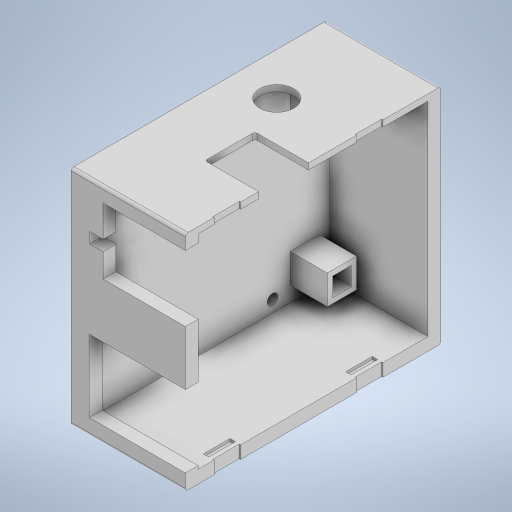
# Autodesk Inventor part: Enclosure_Top_v2
Saved by Autodesk Inventor 2023 (Build 270158030, 158C)
## iProperties
Created: 2023-12-07
Part Number: Enclosure_Top_v2
Material: Generic
Document SubType Name: Sheet Metal
Designer: Fabian
Density: 1 g/cm^3
Sheet Metal Rule: Default_mm
Appearance: Default
Author: Fabian
Autodesk Inventor part; units mm, degrees
ref_plane "YZ Plane" through (0, 0, 0) normal (1, 0, 0) x (0, 1, 0)
ref_plane "XZ Plane" through (0, 0, 0) normal (0, 1, 0) x (-1, 0, 0)
ref_plane "XY Plane" through (0, 0, 0) normal (0, 0, 1) x (1, 0, 0)
sketch "Sketch1" plane through (0, 0, 0) normal (1, 0, 0) x (0, 1, 0)
  line L0 (10.2141, 17.9541) -> (-31.7859, 17.9541)
  line L1 (-31.7859, 17.9541) -> (-31.7859, -30.1559)
  line L2 (-31.7859, -30.1559) -> (10.2141, -30.1559)
  line L3 (10.2141, -30.1559) -> (10.2141, 17.9541)
  point P0 (0, 0)
  dimension "d0" = 42
  dimension "d1" = 48.11
  constraints: 8 end point, 2 parallel, 1 horizontal, 1 perpendicular
  measures "d0" distance of L2.end L1.end
  measures "d1" distance of L1.end L0.end
extrude "BasePlate" add sketch "Sketch1" along normal blind 3
sketch "Sketch3" plane through (3, 0, 0) normal (1, 0, 0) x (0, 0, -1)
  line L0 (30.1559, 10.2141) -> (-17.9541, 10.2141) projected
  line L1 (-17.9541, -31.7859) -> (30.1559, -31.7859) projected
  line L2 (-17.9541, 10.2141) -> (30.1559, 10.2141)
  line L3 (30.1559, 10.2141) -> (30.1559, -31.7859)
  line L4 (30.1559, -31.7859) -> (-17.9541, -31.7859)
  line L5 (-17.9541, -31.7859) -> (-17.9541, 10.2141)
  line L6 (-15.5541, 9.0441) -> (27.7559, 9.0441)
  line L7 (27.7559, 9.0441) -> (27.7559, -29.3859)
  line L8 (27.7559, -29.3859) -> (-15.5541, -29.3859)
  line L9 (-15.5541, -29.3859) -> (-15.5541, 9.0441)
  point P0 (0, 0)
  point P1 (-17.9541, -10.7859)
  dimension "d4" = 1.17
  dimension "d5" = 2.4
  dimension "d6" = 2.4
  dimension "d7" = 2.4
  constraints: 16 end point, 4 parallel, 2 horizontal, 2 perpendicular, 1 midpoint
  measures "d4" distance between parallel lines of L0 L6
  measures "d5" distance between parallel lines of L1 L8
  measures "d6" distance from line of point (-17.954, -10.786) L9
  measures "d7" distance between parallel lines of L3 L7
extrude "Walls" add sketch "Sketch3" along normal blind 18.5
sketch "Sketch4" plane through (21.5, 0, 0) normal (1, 0, 0) x (0, 0, -1)
  line L0 (30.1559, 10.2141) -> (-17.9541, 10.2141) projected
  line L1 (-15.5541, 9.0441) -> (27.7559, 9.0441) projected
  line L2 (-4.1541, 10.2141) -> (5.2459, 10.2141)
  line L3 (5.2459, 10.2141) -> (5.2459, 9.0441)
  line L4 (5.2459, 9.0441) -> (-4.1541, 9.0441)
  line L5 (-4.1541, 9.0441) -> (-4.1541, 10.2141)
  line L6 (-17.9541, 10.2141) -> (-17.9541, -31.7859) projected
  point P0 (0, 0)
  point P1 (-4.1541, 9.6291)
  point P2 (5.2459, 10.2141)
  dimension "d10" = 9.4
  dimension "d11" = 13.8
  constraints: 8 end point, 2 parallel, 2 point on line, 1 horizontal, 1 midpoint, 1 perpendicular
  measures "d10" distance of L3.end L4.end
  measures "d11" distance from line of point (-4.154, 9.629) L6
extrude "USB-C" cut sketch "Sketch4" against normal blind 10.1
sketch "Sketch5" plane through (21.5, 0, 0) normal (1, 0, 0) x (0, 0, -1)
  line L0 (-17.9541, 10.2141) -> (-17.9541, -31.7859) projected
  line L1 (-15.5541, -29.3859) -> (-15.5541, 9.0441) projected
  line L2 (-17.9541, -4.8859) -> (-15.5541, -4.8859)
  line L3 (-15.5541, -4.8859) -> (-15.5541, 7.5141)
  line L4 (-15.5541, 7.5141) -> (-17.9541, 7.5141)
  line L5 (-17.9541, 7.5141) -> (-17.9541, -4.8859)
  line L6 (-4.1541, 10.2141) -> (-17.9541, 10.2141) projected
  point P0 (0, 0)
  point P1 (-16.7541, 7.5141)
  point P2 (-17.9541, 7.5141)
  point P3 (-15.5541, -4.8859)
  dimension "d14" = 12.4
  dimension "d15" = 2.7
  constraints: 8 end point, 2 parallel, 2 point on line, 1 horizontal, 1 midpoint, 1 perpendicular
  measures "d14" distance of L3.end L2.end
  measures "d15" distance from line of L6 point (-16.754, 7.514)
extrude "PowerConnector1" cut sketch "Sketch5" against normal blind 15.5
sketch "Sketch6" plane through (6, 0, 0) normal (1, 0, 0) x (0, 0, -1)
  line L0 (-17.9541, 10.2141) -> (-17.9541, -31.7859) projected
  line L1 (-17.9541, -0.3859) -> (-15.5541, -0.3859)
  line L2 (-15.5541, -0.3859) -> (-15.5541, 1.6141)
  line L3 (-15.5541, 1.6141) -> (-17.9541, 1.6141)
  line L4 (-17.9541, 1.6141) -> (-17.9541, -0.3859)
  line L5 (-17.9541, 7.5141) -> (-15.5541, 7.5141) projected
  point P0 (0, 0)
  dimension "d18" = 2.4
  dimension "d19" = 2
  dimension "d20" = 5.9
  constraints: 8 end point, 2 parallel, 1 horizontal, 1 perpendicular, 1 point on line
  measures "d18" distance of L3.end L2.end
  measures "d19" distance of L1.end L2.end
  measures "d20" distance between parallel lines of L5 L3
extrude "PowerConnector2" cut sketch "Sketch6" against normal blind 2.5
sketch "Sketch8" plane through (21.5, 0, 0) normal (1, 0, 0) x (0, 0, -1)
  line L0 (-17.9541, 10.2141) -> (-17.9541, -31.7859) projected
  line L1 (-15.5541, 9.0441) -> (-15.5541, -29.3859) projected
  line L2 (-17.9541, -28.7859) -> (-15.5541, -28.7859)
  line L3 (-15.5541, -28.7859) -> (-15.5541, -15.1859)
  line L4 (-15.5541, -15.1859) -> (-17.9541, -15.1859)
  line L5 (-17.9541, -15.1859) -> (-17.9541, -28.7859)
  line L6 (-17.9541, -31.7859) -> (30.1559, -31.7859) projected
  point P0 (0, 0)
  dimension "d23" = 13.6
  dimension "d24" = 3
  constraints: 8 end point, 2 parallel, 2 point on line, 1 horizontal, 1 perpendicular
  measures "d23" distance of L3.end L2.end
  measures "d24" distance between parallel lines of L6 L2
extrude "RJ-12" cut sketch "Sketch8" against normal blind 18.1
fillet "Fillet1" radius 0.5 4 edges at (10.75, 10.2141, 17.9541) (10.75, -31.7859, 17.9541) (10.75, 10.2141, -30.1559) (10.75, -31.7859, -30.1559)
sketch "Sketch9" plane through (0, 0, 0) normal (-1, 0, 0) x (0, 0, 1)
  line L0 (-24.8059, -25.5359) -> (-21.3059, -25.5359)
  line L1 (-21.3059, -25.5359) -> (-21.3059, -22.0359)
  line L2 (-21.3059, -22.0359) -> (-24.8059, -22.0359)
  line L3 (-24.8059, -22.0359) -> (-24.8059, -25.5359)
  line L4 (-30.1559, -31.2859) -> (-30.1559, 9.7141) projected
  line L5 (17.4541, -31.7859) -> (-29.6559, -31.7859) projected
  point P0 (0, 0)
  point P1 (-24.8059, -23.7859)
  dimension "d28" = 3.5
  dimension "d29" = 3.5
  dimension "d30" = 5.35
  dimension "d31" = 6.25
  constraints: 8 end point, 2 parallel, 1 horizontal, 1 midpoint, 1 perpendicular
  measures "d28" distance of L2.end L1.end
  measures "d29" distance of L1.end L0.end
  measures "d30" distance from line of L4 point (-24.806, -23.786)
  measures "d31" distance between parallel lines of L5 L0
extrude "ZBButton" cut sketch "Sketch9" against normal blind 3
sketch "Sketch10" plane through (0, 0, 0) normal (-1, 0, 0) x (0, 0, 1)
  line L0 (-24.8059, 0.6641) -> (-21.3059, 0.6641)
  line L1 (-21.3059, 0.6641) -> (-21.3059, 4.1641)
  line L2 (-21.3059, 4.1641) -> (-24.8059, 4.1641)
  line L3 (-24.8059, 4.1641) -> (-24.8059, 0.6641)
  line L4 (-30.1559, -31.2859) -> (-30.1559, 9.7141) projected
  line L5 (-29.6559, 10.2141) -> (17.4541, 10.2141) projected
  point P0 (0, 0)
  point P1 (-24.8059, 2.4141)
  dimension "d34" = 3.5
  dimension "d35" = 3.5
  dimension "d36" = 5.35
  dimension "d37" = 6.05
  constraints: 8 end point, 2 parallel, 1 horizontal, 1 midpoint, 1 perpendicular
  measures "d34" distance of L2.end L1.end
  measures "d35" distance of L1.end L0.end
  measures "d36" distance from line of L4 point (-24.806, 2.414)
  measures "d37" distance between parallel lines of L5 L2
extrude "ResetButton" cut sketch "Sketch10" against normal blind 3
sketch "Sketch11" plane through (3, 0, 0) normal (1, 0, 0) x (0, 0, -1)
  line L0 (25.8059, 5.1641) -> (20.3059, 5.1641)
  line L1 (20.3059, 5.1641) -> (20.3059, -0.3359)
  line L2 (20.3059, -0.3359) -> (25.8059, -0.3359)
  line L3 (25.8059, -0.3359) -> (25.8059, 5.1641)
  line L4 (21.3059, 4.1641) -> (24.8059, 4.1641) projected
  line L5 (24.8059, 4.1641) -> (24.8059, 0.6641) projected
  line L6 (25.8059, -21.0359) -> (20.3059, -21.0359)
  line L7 (20.3059, -21.0359) -> (20.3059, -26.5359)
  line L8 (20.3059, -26.5359) -> (25.8059, -26.5359)
  line L9 (25.8059, -26.5359) -> (25.8059, -21.0359)
  line L10 (24.8059, -22.0359) -> (24.8059, -25.5359) projected
  line L11 (21.3059, -22.0359) -> (24.8059, -22.0359) projected
  line L12 (24.8059, 0.6641) -> (21.3059, 0.6641) projected
  line L13 (24.8059, 4.1641) -> (21.3059, 4.1641)
  line L14 (21.3059, 4.1641) -> (21.3059, 0.6641)
  line L15 (21.3059, 0.6641) -> (24.8059, 0.6641)
  line L16 (24.8059, 0.6641) -> (24.8059, 4.1641)
  line L17 (21.3059, -25.5359) -> (21.3059, -22.0359) projected
  line L18 (24.8059, -22.0359) -> (21.3059, -22.0359)
  line L19 (21.3059, -22.0359) -> (21.3059, -25.5359)
  line L20 (21.3059, -25.5359) -> (24.8059, -25.5359)
  line L21 (24.8059, -25.5359) -> (24.8059, -22.0359)
  point P0 (0, 0)
  point P1 (23.0559, -22.0359)
  dimension "d40" = 5.5
  dimension "d41" = 5.5
  dimension "d42" = 1
  dimension "d43" = 1
  dimension "d44" = 5.5
  dimension "d45" = 5.5
  dimension "d46" = 1
  dimension "d47" = 1
  constraints: 32 end point, 8 parallel, 4 horizontal, 4 perpendicular, 1 midpoint
  measures "d40" distance of L2.end L1.end
  measures "d41" distance of L1.end L0.end
  measures "d42" distance between parallel lines of L4 L0
  measures "d43" distance between parallel lines of L3 L5
  measures "d44" distance of L8.end L7.end
  measures "d45" distance of L7.end L6.end
  measures "d46" distance between parallel lines of L9 L10
  measures "d47" distance from line of point (23.056, -22.036) L6
extrude "ButtonFuehrung" add sketch "Sketch11" along normal blind 7
sketch "Sketch12" plane through (0, 0, 0) normal (-1, 0, 0) x (0, 0, 1)
  circle A0 centre (-16.9559, -27.1859) radius 1
  line L0 (17.4541, -31.7859) -> (-29.6559, -31.7859) projected
  line L1 (-30.1559, -31.2859) -> (-30.1559, 9.7141) projected
  point P0 (0, 0)
  dimension "d50" = 2
  dimension "d51" = 4.6
  dimension "d52" = 13.2
  constraints: 1 centre point
  measures "d50" diameter of A0
  measures "d51" distance from line of L0 A0.centre
  measures "d52" distance from line of L1 A0.centre
extrude "LED" cut sketch "Sketch12" against normal blind 3
sketch "Sketch13" plane through (11.4, 10.2141, 4.1541) normal (0, 1, 0) x (1, 0, 0)
  circle A0 centre (-3.4, 16.91) radius 3.2
  line L0 (-11.4, 33.81) -> (-11.4, -13.3) projected
  line L1 (10.1, 34.31) -> (-11.4, 34.31) projected
  point P0 (-11.4, 4.1541)
  dimension "d55" = 6.4
  dimension "d56" = 8
  dimension "d57" = 17.4
  constraints: 1 centre point
  measures "d55" diameter of A0
  measures "d56" distance from line of L0 A0.centre
  measures "d57" distance from line of L1 A0.centre
extrude "Antenna" cut sketch "Sketch13" against normal blind 2
sketch "Sketch14" plane through (3, 9.0441, -27.7559) normal (0, -1, 0) x (1, 0, 0)
  line L0 (17.5, 40.31) -> (16.5, 40.31)
  line L1 (16.5, 40.31) -> (16.5, 35.31)
  line L2 (16.5, 35.31) -> (17.5, 35.31)
  line L3 (17.5, 35.31) -> (17.5, 40.31)
  line L4 (18.5, 43.31) -> (18.5, 31.91) projected
  point P0 (-3, 27.7559)
  point P1 (17.5, 37.81)
  dimension "d60" = 1
  dimension "d61" = 5
  dimension "d62" = 1
  dimension "d63" = 5.5
  constraints: 8 end point, 2 parallel, 1 horizontal, 1 midpoint, 1 perpendicular
  measures "d60" distance of L2.end L1.end
  measures "d61" distance of L1.end L0.end
  measures "d62" distance between parallel lines of L4 L3
  measures "d63" vertical distance of L4.start point (17.5, 37.81)
extrude "Extrusion12" cut sketch "Sketch14" against normal blind 0.5
sketch "Sketch15" plane through (3, 9.0441, -27.7559) normal (0, -1, 0) x (1, 0, 0)
  line L0 (17.5, 13.5) -> (16.5, 13.5)
  line L1 (16.5, 13.5) -> (16.5, 8.5)
  line L2 (16.5, 8.5) -> (17.5, 8.5)
  line L3 (17.5, 8.5) -> (17.5, 13.5)
  line L4 (18.5, 22.51) -> (18.5, 0) projected
  line L5 (0, 0) -> (18.5, 0) projected
  point P0 (-3, 27.7559)
  point P1 (17.5, 11)
  dimension "d66" = 1
  dimension "d67" = 5
  dimension "d68" = 1
  dimension "d69" = 11
  constraints: 8 end point, 2 parallel, 1 horizontal, 1 midpoint, 1 perpendicular
  measures "d66" distance of L2.end L1.end
  measures "d67" distance of L1.end L0.end
  measures "d68" distance from line of L4 point (17.5, 11)
  measures "d69" distance from line of L5 point (17.5, 11)
extrude "Extrusion13" cut sketch "Sketch15" against normal blind 0.5
sketch "Sketch16" plane through (3, -29.3859, 15.5541) normal (0, 1, 0) x (1, 0, 0)
  line L0 (17.5, 8) -> (16.5, 8)
  line L1 (16.5, 8) -> (16.5, 3)
  line L2 (16.5, 3) -> (17.5, 3)
  line L3 (17.5, 3) -> (17.5, 8)
  line L4 (18.5, 43.31) -> (18.5, 0) projected
  line L5 (0, 0) -> (18.5, 0) projected
  point P0 (-3, 15.5541)
  point P1 (17.5, 5.5)
  dimension "d72" = 1
  dimension "d73" = 5
  dimension "d74" = 1
  dimension "d75" = 5.5
  constraints: 8 end point, 2 parallel, 1 horizontal, 1 midpoint, 1 perpendicular
  measures "d72" distance of L2.end L1.end
  measures "d73" distance of L1.end L0.end
  measures "d74" distance between parallel lines of L4 L3
  measures "d75" distance from line of L5 point (17.5, 5.5)
extrude "Extrusion14" cut sketch "Sketch16" against normal blind 0.5
sketch "Sketch17" plane through (3, -29.3859, 15.5541) normal (0, 1, 0) x (1, 0, 0)
  line L0 (17.5, 34.81) -> (16.5, 34.81)
  line L1 (16.5, 34.81) -> (16.5, 29.81)
  line L2 (16.5, 29.81) -> (17.5, 29.81)
  line L3 (17.5, 29.81) -> (17.5, 34.81)
  line L4 (18.5, 43.31) -> (18.5, 0) projected
  line L5 (0, 43.31) -> (18.5, 43.31) projected
  point P0 (-3, 15.5541)
  point P1 (17.5, 32.31)
  dimension "d78" = 1
  dimension "d79" = 5
  dimension "d80" = 1
  dimension "d81" = 11
  constraints: 8 end point, 2 parallel, 1 horizontal, 1 midpoint, 1 perpendicular
  measures "d78" distance of L2.end L1.end
  measures "d79" distance of L1.end L0.end
  measures "d80" distance between parallel lines of L4 L3
  measures "d81" distance from line of L5 point (17.5, 32.31)
extrude "Extrusion15" cut sketch "Sketch17" against normal blind 0.5
fillet "Fillet2" radius 0.5 2 edges at (11.4, 9.6291, -5.2459) (11.4, 9.6291, 4.1541)
sketch "Sketch18" plane through (0, 0, 0) normal (-1, 0, 0) x (0, 0, 1)
  line L0 (-25.0559, 8.7746) -> (-25.0559, -4.7256) construction
  line L1 (-25.0559, -4.7256) -> (-29.2477, -4.7256) construction
  line L2 (-29.2477, -4.7256) -> (-29.2477, 8.7746) construction
  line L3 (-29.2477, 8.7746) -> (-25.0559, 8.7746) construction
  line L4 (-25.0559, -16.0398) -> (-25.0559, -32.4133) construction
  line L5 (-25.0559, -32.4133) -> (-30.1806, -32.4133) construction
  line L6 (-30.1806, -32.4133) -> (-30.1806, -16.0398) construction
  line L7 (-30.1806, -16.0398) -> (-25.0559, -16.0398) construction
  line L8 (-24.8059, -25.5359) -> (-24.8059, -22.0359) projected
  line L9 (-24.8059, 0.6641) -> (-24.8059, 4.1641) projected
  line L10 (-28.5559, 5.7114) -> (-28.5559, 6.3155)
  line L11 (-28.5559, 6.3155) -> (-27.1633, 7.4217)
  line L12 (-27.1633, 7.4217) -> (-27.1633, 7.9549)
  line L13 (-27.1633, 7.9549) -> (-28.5559, 7.9549)
  line L14 (-28.5559, 7.9549) -> (-28.5559, 8.42)
  line L15 (-28.5559, 8.42) -> (-25.0559, 8.42)
  line L16 (-25.0559, 8.42) -> (-25.0559, 7.5181)
  spline S0 degree 2 poles (-25.0559, 7.5181) (-25.0559, 7.2174) (-25.1212, 6.8119) (-25.2403, 6.6275) knots 0 0 0 1 2 2 2
  spline S1 degree 2 poles (-25.2403, 6.6275) (-25.3594, 6.4431) (-25.731, 6.2304) (-26.0061, 6.2304) knots 0 0 0 1 2 2 2
  spline S2 degree 2 poles (-26.0061, 6.2304) (-26.389, 6.2304) (-26.908, 6.6218) (-27.0328, 6.9565) knots 0 0 0 1 2 2 2
  line L17 (-27.0328, 6.9565) -> (-28.5559, 5.7114)
  spline S3 degree 2 poles (-26.043, 6.7154) (-25.8898, 6.7154) (-25.6544, 6.8232) (-25.5778, 6.9367) knots 0 0 0 1 2 2 2
  spline S4 degree 2 poles (-25.5778, 6.9367) (-25.5126, 7.0359) (-25.4587, 7.2997) (-25.4587, 7.4926) knots 0 0 0 1 2 2 2
  line L18 (-25.4587, 7.4926) -> (-25.4587, 7.9549)
  line L19 (-25.4587, 7.9549) -> (-26.7747, 7.9549)
  line L20 (-26.7747, 7.9549) -> (-26.7747, 7.5465)
  spline S5 degree 2 poles (-26.7747, 7.5465) (-26.7747, 7.3451) (-26.7038, 7.0246) (-26.5932, 6.914) knots 0 0 0 1 2 2 2
  spline S6 degree 2 poles (-26.5932, 6.914) (-26.4968, 6.8119) (-26.2245, 6.7154) (-26.043, 6.7154) knots 0 0 0 1 2 2 2
  spline S7 degree 2 poles (-28.6155, 4.3272) (-28.6155, 4.9569) (-27.9093, 5.649) (-27.2569, 5.649) knots 0 0 0 1 2 2 2
  spline S8 degree 2 poles (-27.2569, 5.649) (-26.6159, 5.649) (-25.8558, 4.9768) (-25.8558, 4.435) knots 0 0 0 1 2 2 2
  spline S9 degree 2 poles (-25.8558, 4.435) (-25.8558, 4.1911) (-25.9976, 3.8139) (-26.1479, 3.6749) knots 0 0 0 1 2 2 2
  spline S10 degree 2 poles (-26.1479, 3.6749) (-26.2982, 3.5331) (-26.7322, 3.3828) (-27.047, 3.3828) knots 0 0 0 1 2 2 2
  line L21 (-27.047, 3.3828) -> (-27.2881, 3.3828)
  line L22 (-27.2881, 3.3828) -> (-27.2881, 5.2008)
  spline S11 degree 2 poles (-27.2881, 5.2008) (-27.7448, 5.2008) (-28.2298, 4.7414) (-28.2298, 4.3329) knots 0 0 0 1 2 2 2
  spline S12 degree 2 poles (-28.2298, 4.3329) (-28.2298, 4.1883) (-28.1645, 3.9075) (-28.1135, 3.794) knots 0 0 0 1 2 2 2
  spline S13 degree 2 poles (-28.1135, 3.794) (-28.0568, 3.6749) (-27.9575, 3.5104) (-27.9121, 3.4565) knots 0 0 0 1 2 2 2
  line L23 (-27.9121, 3.4565) -> (-27.9121, 3.431)
  line L24 (-27.9121, 3.431) -> (-28.3943, 3.431)
  spline S14 degree 2 poles (-28.3943, 3.431) (-28.4255, 3.5076) (-28.5162, 3.7401) (-28.5418, 3.8309) knots 0 0 0 1 2 2 2
  spline S15 degree 2 poles (-28.5418, 3.8309) (-28.5786, 3.9585) (-28.6155, 4.1684) (-28.6155, 4.3272) knots 0 0 0 1 2 2 2
  spline S16 degree 2 poles (-26.9506, 3.8139) (-26.7719, 3.8196) (-26.511, 3.8933) (-26.423, 3.9642) knots 0 0 0 1 2 2 2
  spline S17 degree 2 poles (-26.423, 3.9642) (-26.3238, 4.0408) (-26.2188, 4.2819) (-26.2188, 4.4606) knots 0 0 0 1 2 2 2
  spline S18 degree 2 poles (-26.2188, 4.4606) (-26.2188, 4.6364) (-26.3238, 4.8832) (-26.4259, 4.9853) knots 0 0 0 1 2 2 2
  spline S19 degree 2 poles (-26.4259, 4.9853) (-26.5308, 5.0845) (-26.7833, 5.1867) (-26.9506, 5.2008) knots 0 0 0 1 2 2 2
  line L25 (-26.9506, 5.2008) -> (-26.9506, 3.8139)
  spline S20 degree 2 poles (-28.6183, 2.2255) (-28.6183, 2.4893) (-28.4765, 2.946) (-28.3971, 3.0963) knots 0 0 0 1 2 2 2
  line L26 (-28.3971, 3.0963) -> (-27.9008, 3.0963)
  line L27 (-27.9008, 3.0963) -> (-27.9008, 3.0736)
  spline S21 degree 2 poles (-27.9008, 3.0736) (-27.9461, 3.0169) (-28.0539, 2.8637) (-28.1135, 2.7361) knots 0 0 0 1 2 2 2
  spline S22 degree 2 poles (-28.1135, 2.7361) (-28.1674, 2.6255) (-28.2468, 2.3532) (-28.2468, 2.2085) knots 0 0 0 1 2 2 2
  spline S23 degree 2 poles (-28.2468, 2.2085) (-28.2468, 2.1036) (-28.1986, 1.8625) (-28.1589, 1.8058) knots 0 0 0 1 2 2 2
  spline S24 degree 2 poles (-28.1589, 1.8058) (-28.105, 1.7235) (-27.983, 1.6498) (-27.8582, 1.6498) knots 0 0 0 1 2 2 2
  spline S25 degree 2 poles (-27.8582, 1.6498) (-27.7022, 1.6498) (-27.5405, 1.82) (-27.4867, 2.0384) knots 0 0 0 1 2 2 2
  spline S26 degree 2 poles (-27.4867, 2.0384) (-27.4668, 2.1234) (-27.4101, 2.3957) (-27.3789, 2.512) knots 0 0 0 1 2 2 2
  spline S27 degree 2 poles (-27.3789, 2.512) (-27.2909, 2.8127) (-26.9279, 3.0849) (-26.6698, 3.0849) knots 0 0 0 1 2 2 2
  spline S28 degree 2 poles (-26.6698, 3.0849) (-26.3124, 3.0849) (-25.8671, 2.5489) (-25.8671, 2.1064) knots 0 0 0 1 2 2 2
  spline S29 degree 2 poles (-25.8671, 2.1064) (-25.8671, 1.888) (-25.9749, 1.4456) (-26.0572, 1.2952) knots 0 0 0 1 2 2 2
  line L28 (-26.0572, 1.2952) -> (-26.5308, 1.2952)
  line L29 (-26.5308, 1.2952) -> (-26.5308, 1.3179)
  spline S30 degree 2 poles (-26.5308, 1.3179) (-26.3947, 1.4881) (-26.2387, 1.9022) (-26.2387, 2.1149) knots 0 0 0 1 2 2 2
  spline S31 degree 2 poles (-26.2387, 2.1149) (-26.2387, 2.3333) (-26.423, 2.634) (-26.6074, 2.634) knots 0 0 0 1 2 2 2
  spline S32 degree 2 poles (-26.6074, 2.634) (-26.7747, 2.634) (-26.9364, 2.4553) (-26.9875, 2.2567) knots 0 0 0 1 2 2 2
  spline S33 degree 2 poles (-26.9875, 2.2567) (-27.013, 2.1603) (-27.064, 1.9164) (-27.0952, 1.7831) knots 0 0 0 1 2 2 2
  spline S34 degree 2 poles (-27.0952, 1.7831) (-27.169, 1.4938) (-27.5065, 1.1988) (-27.7986, 1.1988) knots 0 0 0 1 2 2 2
  spline S35 degree 2 poles (-27.7986, 1.1988) (-27.9688, 1.1988) (-28.2695, 1.3321) (-28.3801, 1.4626) knots 0 0 0 1 2 2 2
  spline S36 degree 2 poles (-28.3801, 1.4626) (-28.4964, 1.6016) (-28.6183, 1.9561) (-28.6183, 2.2255) knots 0 0 0 1 2 2 2
  spline S37 degree 2 poles (-28.6155, -0.3527) (-28.6155, 0.277) (-27.9093, 0.9691) (-27.2569, 0.9691) knots 0 0 0 1 2 2 2
  spline S38 degree 2 poles (-27.2569, 0.9691) (-26.6159, 0.9691) (-25.8558, 0.2969) (-25.8558, -0.2449) knots 0 0 0 1 2 2 2
  spline S39 degree 2 poles (-25.8558, -0.2449) (-25.8558, -0.4888) (-25.9976, -0.866) (-26.1479, -1.005) knots 0 0 0 1 2 2 2
  spline S40 degree 2 poles (-26.1479, -1.005) (-26.2982, -1.1468) (-26.7322, -1.2971) (-27.047, -1.2971) knots 0 0 0 1 2 2 2
  line L30 (-27.047, -1.2971) -> (-27.2881, -1.2971)
  line L31 (-27.2881, -1.2971) -> (-27.2881, 0.5209)
  spline S41 degree 2 poles (-27.2881, 0.5209) (-27.7448, 0.5209) (-28.2298, 0.0614) (-28.2298, -0.347) knots 0 0 0 1 2 2 2
  spline S42 degree 2 poles (-28.2298, -0.347) (-28.2298, -0.4916) (-28.1645, -0.7724) (-28.1135, -0.8859) knots 0 0 0 1 2 2 2
  spline S43 degree 2 poles (-28.1135, -0.8859) (-28.0568, -1.005) (-27.9575, -1.1695) (-27.9121, -1.2234) knots 0 0 0 1 2 2 2
  line L32 (-27.9121, -1.2234) -> (-27.9121, -1.2489)
  line L33 (-27.9121, -1.2489) -> (-28.3943, -1.2489)
  spline S44 degree 2 poles (-28.3943, -1.2489) (-28.4255, -1.1723) (-28.5162, -0.9398) (-28.5418, -0.849) knots 0 0 0 1 2 2 2
  spline S45 degree 2 poles (-28.5418, -0.849) (-28.5786, -0.7214) (-28.6155, -0.5115) (-28.6155, -0.3527) knots 0 0 0 1 2 2 2
  spline S46 degree 2 poles (-26.9506, -0.866) (-26.7719, -0.8604) (-26.511, -0.7866) (-26.423, -0.7157) knots 0 0 0 1 2 2 2
  spline S47 degree 2 poles (-26.423, -0.7157) (-26.3238, -0.6391) (-26.2188, -0.398) (-26.2188, -0.2193) knots 0 0 0 1 2 2 2
  spline S48 degree 2 poles (-26.2188, -0.2193) (-26.2188, -0.0435) (-26.3238, 0.2033) (-26.4259, 0.3054) knots 0 0 0 1 2 2 2
  spline S49 degree 2 poles (-26.4259, 0.3054) (-26.5308, 0.4046) (-26.7833, 0.5067) (-26.9506, 0.5209) knots 0 0 0 1 2 2 2
  line L34 (-26.9506, 0.5209) -> (-26.9506, -0.866)
  spline S50 degree 2 poles (-28.607, -2.5394) (-28.607, -2.1792) (-28.1957, -1.7736) (-27.7504, -1.7736) knots 0 0 0 1 2 2 2
  line L35 (-27.7504, -1.7736) -> (-26.2954, -1.7736)
  line L36 (-26.2954, -1.7736) -> (-26.2954, -1.4758)
  line L37 (-26.2954, -1.4758) -> (-25.9295, -1.4758)
  line L38 (-25.9295, -1.4758) -> (-25.9295, -1.7736)
  line L39 (-25.9295, -1.7736) -> (-25.1751, -1.7736)
  line L40 (-25.1751, -1.7736) -> (-25.1751, -2.2161)
  line L41 (-25.1751, -2.2161) -> (-25.9295, -2.2161)
  line L42 (-25.9295, -2.2161) -> (-25.9295, -3.0301)
  line L43 (-25.9295, -3.0301) -> (-26.2954, -3.0301)
  line L44 (-26.2954, -3.0301) -> (-26.2954, -2.2161)
  line L45 (-26.2954, -2.2161) -> (-27.5462, -2.2161)
  spline S51 degree 2 poles (-27.5462, -2.2161) (-27.7448, -2.2161) (-27.9632, -2.2303) (-28.0568, -2.2785) knots 0 0 0 1 2 2 2
  spline S52 degree 2 poles (-28.0568, -2.2785) (-28.139, -2.3182) (-28.2213, -2.4969) (-28.2213, -2.6501) knots 0 0 0 1 2 2 2
  spline S53 degree 2 poles (-28.2213, -2.6501) (-28.2213, -2.7578) (-28.156, -2.9592) (-28.1362, -3.0046) knots 0 0 0 1 2 2 2
  line L46 (-28.1362, -3.0046) -> (-28.1362, -3.0301)
  line L47 (-28.1362, -3.0301) -> (-28.5333, -3.0301)
  spline S54 degree 2 poles (-28.5333, -3.0301) (-28.5673, -2.9053) (-28.607, -2.6501) (-28.607, -2.5394) knots 0 0 0 1 2 2 2
  line L48 (-28.5786, -18.6265) -> (-28.5786, -16.1816)
  line L49 (-28.5786, -16.1816) -> (-28.1447, -16.1816)
  line L50 (-28.1447, -16.1816) -> (-25.4927, -18.0535)
  line L51 (-25.4927, -18.0535) -> (-25.4927, -16.2667)
  line L52 (-25.4927, -16.2667) -> (-25.0786, -16.2667)
  line L53 (-25.0786, -16.2667) -> (-25.0786, -18.5783)
  line L54 (-25.0786, -18.5783) -> (-25.4984, -18.5783)
  line L55 (-25.4984, -18.5783) -> (-28.1645, -16.6864)
  line L56 (-28.1645, -16.6864) -> (-28.1645, -18.6265)
  line L57 (-28.1645, -18.6265) -> (-28.5786, -18.6265)
  line L58 (-28.5786, -19.5029) -> (-28.5786, -19.0604)
  line L59 (-28.5786, -19.0604) -> (-25.9522, -19.0604)
  line L60 (-25.9522, -19.0604) -> (-25.9522, -19.5029)
  line L61 (-25.9522, -19.5029) -> (-28.5786, -19.5029)
  line L62 (-25.5154, -19.5341) -> (-25.5154, -19.0321)
  line L63 (-25.5154, -19.0321) -> (-25.0559, -19.0321)
  line L64 (-25.0559, -19.0321) -> (-25.0559, -19.5341)
  line L65 (-25.0559, -19.5341) -> (-25.5154, -19.5341)
  spline S55 degree 2 poles (-28.9984, -20.246) (-29.0183, -20.2914) (-29.0807, -20.4644) (-29.1062, -20.575) knots 0 0 0 1 2 2 2
  spline S56 degree 2 poles (-29.1062, -20.575) (-29.1374, -20.697) (-29.1743, -20.904) (-29.1743, -21.026) knots 0 0 0 1 2 2 2
  spline S57 degree 2 poles (-29.1743, -21.026) (-29.1743, -21.2302) (-29.0665, -21.5138) (-28.97, -21.5933) knots 0 0 0 1 2 2 2
  spline S58 degree 2 poles (-28.97, -21.5933) (-28.8736, -21.6698) (-28.6212, -21.7294) (-28.4595, -21.7294) knots 0 0 0 1 2 2 2
  line L66 (-28.4595, -21.7294) -> (-28.2298, -21.7294)
  spline S59 degree 2 poles (-28.2298, -21.7294) (-28.3858, -21.5507) (-28.5333, -21.2075) (-28.5333, -20.9494) knots 0 0 0 1 2 2 2
  spline S60 degree 2 poles (-28.5333, -20.9494) (-28.5333, -20.5013) (-27.8667, -19.9709) (-27.2399, -19.9709) knots 0 0 0 1 2 2 2
  spline S61 degree 2 poles (-27.2399, -19.9709) (-26.9137, -19.9709) (-26.4089, -20.1552) (-26.2302, -20.3084) knots 0 0 0 1 2 2 2
  spline S62 degree 2 poles (-26.2302, -20.3084) (-26.0628, -20.4559) (-25.8785, -20.8615) (-25.8785, -21.077) knots 0 0 0 1 2 2 2
  spline S63 degree 2 poles (-25.8785, -21.077) (-25.8785, -21.2813) (-25.9749, -21.5791) (-26.0628, -21.7294) knots 0 0 0 1 2 2 2
  line L67 (-26.0628, -21.7294) -> (-25.9522, -21.7549)
  line L68 (-25.9522, -21.7549) -> (-25.9522, -22.1719)
  line L69 (-25.9522, -22.1719) -> (-28.278, -22.1719)
  spline S64 degree 2 poles (-28.278, -22.1719) (-28.9474, -22.1719) (-29.5713, -21.5904) (-29.5713, -20.992) knots 0 0 0 1 2 2 2
  spline S65 degree 2 poles (-29.5713, -20.992) (-29.5713, -20.7991) (-29.5089, -20.3963) (-29.4579, -20.2233) knots 0 0 0 1 2 2 2
  line L70 (-29.4579, -20.2233) -> (-28.9984, -20.2233)
  line L71 (-28.9984, -20.2233) -> (-28.9984, -20.246)
  line L72 (-27.8667, -21.7294) -> (-26.423, -21.7294)
  spline S66 degree 2 poles (-26.423, -21.7294) (-26.3436, -21.5649) (-26.2756, -21.2869) (-26.2756, -21.148) knots 0 0 0 1 2 2 2
  spline S67 degree 2 poles (-26.2756, -21.148) (-26.2756, -20.8133) (-26.7691, -20.4275) (-27.2314, -20.4275) knots 0 0 0 1 2 2 2
  spline S68 degree 2 poles (-27.2314, -20.4275) (-27.6682, -20.4275) (-28.1248, -20.7197) (-28.1248, -21.0487) knots 0 0 0 1 2 2 2
  spline S69 degree 2 poles (-28.1248, -21.0487) (-28.1248, -21.2217) (-27.9887, -21.5847) (-27.8667, -21.7294) knots 0 0 0 1 2 2 2
  spline S70 degree 2 poles (-27.5037, -25.2209) (-27.7646, -25.2209) (-28.1645, -25.0223) (-28.295, -24.8578) knots 0 0 0 1 2 2 2
  spline S71 degree 2 poles (-28.295, -24.8578) (-28.4482, -24.6593) (-28.5786, -24.2083) (-28.5786, -23.851) knots 0 0 0 1 2 2 2
  line L73 (-28.5786, -23.851) -> (-28.5786, -22.8469)
  line L74 (-28.5786, -22.8469) -> (-25.0786, -22.8469)
  line L75 (-25.0786, -22.8469) -> (-25.0786, -23.7744)
  spline S72 degree 2 poles (-25.0786, -23.7744) (-25.0786, -24.1488) (-25.1268, -24.5232) (-25.2204, -24.6933) knots 0 0 0 1 2 2 2
  spline S73 degree 2 poles (-25.2204, -24.6933) (-25.3197, -24.8834) (-25.6459, -25.0564) (-25.8671, -25.0564) knots 0 0 0 1 2 2 2
  spline S74 degree 2 poles (-25.8671, -25.0564) (-26.1139, -25.0564) (-26.5053, -24.7954) (-26.6159, -24.5657) knots 0 0 0 1 2 2 2
  line L76 (-26.6159, -24.5657) -> (-26.6329, -24.5657)
  spline S75 degree 2 poles (-26.6329, -24.5657) (-26.718, -24.8777) (-27.169, -25.2209) (-27.5037, -25.2209) knots 0 0 0 1 2 2 2
  spline S76 degree 2 poles (-27.5235, -24.7359) (-27.325, -24.7359) (-27.0697, -24.6224) (-26.979, -24.4523) knots 0 0 0 1 2 2 2
  spline S77 degree 2 poles (-26.979, -24.4523) (-26.9222, -24.3416) (-26.8882, -24.0807) (-26.8882, -23.8396) knots 0 0 0 1 2 2 2
  line L77 (-26.8882, -23.8396) -> (-26.8882, -23.3121)
  line L78 (-26.8882, -23.3121) -> (-28.1815, -23.3121)
  line L79 (-28.1815, -23.3121) -> (-28.1815, -23.6893)
  spline S78 degree 2 poles (-28.1815, -23.6893) (-28.1815, -23.9956) (-28.1248, -24.3473) (-28.0341, -24.4835) knots 0 0 0 1 2 2 2
  spline S79 degree 2 poles (-28.0341, -24.4835) (-27.9405, -24.6139) (-27.7079, -24.7359) (-27.5235, -24.7359) knots 0 0 0 1 2 2 2
  spline S80 degree 2 poles (-25.9324, -24.5714) (-25.8076, -24.5714) (-25.6204, -24.4863) (-25.5665, -24.3927) knots 0 0 0 1 2 2 2
  spline S81 degree 2 poles (-25.5665, -24.3927) (-25.5041, -24.2792) (-25.4757, -24.0041) (-25.4757, -23.7574) knots 0 0 0 1 2 2 2
  line L80 (-25.4757, -23.7574) -> (-25.4757, -23.3121)
  line L81 (-25.4757, -23.3121) -> (-26.4996, -23.3121)
  line L82 (-26.4996, -23.3121) -> (-26.4996, -23.8396)
  spline S82 degree 2 poles (-26.4996, -23.8396) (-26.4996, -24.058) (-26.4542, -24.2651) (-26.3833, -24.3757) knots 0 0 0 1 2 2 2
  spline S83 degree 2 poles (-26.3833, -24.3757) (-26.3153, -24.4835) (-26.0969, -24.5714) (-25.9324, -24.5714) knots 0 0 0 1 2 2 2
  spline S84 degree 2 poles (-28.6382, -26.7894) (-28.6382, -26.1597) (-27.932, -25.4676) (-27.2796, -25.4676) knots 0 0 0 1 2 2 2
  spline S85 degree 2 poles (-27.2796, -25.4676) (-26.6386, -25.4676) (-25.8785, -26.1399) (-25.8785, -26.6816) knots 0 0 0 1 2 2 2
  spline S86 degree 2 poles (-25.8785, -26.6816) (-25.8785, -26.9255) (-26.0203, -27.3027) (-26.1706, -27.4417) knots 0 0 0 1 2 2 2
  spline S87 degree 2 poles (-26.1706, -27.4417) (-26.3209, -27.5835) (-26.7549, -27.7339) (-27.0697, -27.7339) knots 0 0 0 1 2 2 2
  line L83 (-27.0697, -27.7339) -> (-27.3108, -27.7339)
  line L84 (-27.3108, -27.7339) -> (-27.3108, -25.9158)
  spline S88 degree 2 poles (-27.3108, -25.9158) (-27.7674, -25.9158) (-28.2525, -26.3753) (-28.2525, -26.7837) knots 0 0 0 1 2 2 2
  spline S89 degree 2 poles (-28.2525, -26.7837) (-28.2525, -26.9283) (-28.1872, -27.2091) (-28.1362, -27.3226) knots 0 0 0 1 2 2 2
  spline S90 degree 2 poles (-28.1362, -27.3226) (-28.0794, -27.4417) (-27.9802, -27.6062) (-27.9348, -27.6601) knots 0 0 0 1 2 2 2
  line L85 (-27.9348, -27.6601) -> (-27.9348, -27.6856)
  line L86 (-27.9348, -27.6856) -> (-28.417, -27.6856)
  spline S91 degree 2 poles (-28.417, -27.6856) (-28.4482, -27.6091) (-28.5389, -27.3765) (-28.5645, -27.2857) knots 0 0 0 1 2 2 2
  spline S92 degree 2 poles (-28.5645, -27.2857) (-28.6013, -27.1581) (-28.6382, -26.9482) (-28.6382, -26.7894) knots 0 0 0 1 2 2 2
  spline S93 degree 2 poles (-26.9733, -27.3027) (-26.7946, -27.2971) (-26.5337, -27.2233) (-26.4457, -27.1524) knots 0 0 0 1 2 2 2
  spline S94 degree 2 poles (-26.4457, -27.1524) (-26.3465, -27.0758) (-26.2415, -26.8347) (-26.2415, -26.6561) knots 0 0 0 1 2 2 2
  spline S95 degree 2 poles (-26.2415, -26.6561) (-26.2415, -26.4802) (-26.3465, -26.2335) (-26.4486, -26.1313) knots 0 0 0 1 2 2 2
  spline S96 degree 2 poles (-26.4486, -26.1313) (-26.5535, -26.0321) (-26.8059, -25.93) (-26.9733, -25.9158) knots 0 0 0 1 2 2 2
  line L87 (-26.9733, -25.9158) -> (-26.9733, -27.3027)
  spline S97 degree 2 poles (-28.6382, -29.3222) (-28.6382, -28.6925) (-27.932, -28.0005) (-27.2796, -28.0005) knots 0 0 0 1 2 2 2
  spline S98 degree 2 poles (-27.2796, -28.0005) (-26.6386, -28.0005) (-25.8785, -28.6727) (-25.8785, -29.2144) knots 0 0 0 1 2 2 2
  spline S99 degree 2 poles (-25.8785, -29.2144) (-25.8785, -29.4583) (-26.0203, -29.8356) (-26.1706, -29.9745) knots 0 0 0 1 2 2 2
  spline S100 degree 2 poles (-26.1706, -29.9745) (-26.3209, -30.1164) (-26.7549, -30.2667) (-27.0697, -30.2667) knots 0 0 0 1 2 2 2
  line L88 (-27.0697, -30.2667) -> (-27.3108, -30.2667)
  line L89 (-27.3108, -30.2667) -> (-27.3108, -28.4486)
  spline S101 degree 2 poles (-27.3108, -28.4486) (-27.7674, -28.4486) (-28.2525, -28.9081) (-28.2525, -29.3165) knots 0 0 0 1 2 2 2
  spline S102 degree 2 poles (-28.2525, -29.3165) (-28.2525, -29.4612) (-28.1872, -29.742) (-28.1362, -29.8554) knots 0 0 0 1 2 2 2
  spline S103 degree 2 poles (-28.1362, -29.8554) (-28.0794, -29.9745) (-27.9802, -30.139) (-27.9348, -30.1929) knots 0 0 0 1 2 2 2
  line L90 (-27.9348, -30.1929) -> (-27.9348, -30.2185)
  line L91 (-27.9348, -30.2185) -> (-28.417, -30.2185)
  spline S104 degree 2 poles (-28.417, -30.2185) (-28.4482, -30.1419) (-28.5389, -29.9093) (-28.5645, -29.8185) knots 0 0 0 1 2 2 2
  spline S105 degree 2 poles (-28.5645, -29.8185) (-28.6013, -29.6909) (-28.6382, -29.481) (-28.6382, -29.3222) knots 0 0 0 1 2 2 2
  spline S106 degree 2 poles (-26.9733, -29.8356) (-26.7946, -29.8299) (-26.5337, -29.7561) (-26.4457, -29.6852) knots 0 0 0 1 2 2 2
  spline S107 degree 2 poles (-26.4457, -29.6852) (-26.3465, -29.6087) (-26.2415, -29.3676) (-26.2415, -29.1889) knots 0 0 0 1 2 2 2
  spline S108 degree 2 poles (-26.2415, -29.1889) (-26.2415, -29.013) (-26.3465, -28.7663) (-26.4486, -28.6642) knots 0 0 0 1 2 2 2
  spline S109 degree 2 poles (-26.4486, -28.6642) (-26.5535, -28.5649) (-26.8059, -28.4628) (-26.9733, -28.4486) knots 0 0 0 1 2 2 2
  line L92 (-26.9733, -28.4486) -> (-26.9733, -29.8356)
  point P0 (0, 0)
  point P1 (-25.0559, 2.0245)
  dimension "d85" = 0.25
  dimension "d86" = 0.25
  constraints: 1 midpoint, 4 other
  measures "d85" distance between parallel lines of L4 L8
  measures "d86" distance from line of L9 point (-25.056, 2.024)
emboss "Emboss1" sketch "Sketch18" operation cut depth 1 direction (1, 0, 0)
sketch "Sketch23" plane through (3, -29.3859, 15.5541) normal (0, 1, 0) x (1, 0, 0)
  line L0 (18.5, 43.31) -> (18.5, 0) projected
  line L1 (18.5, 3) -> (18.25, 3)
  line L2 (18.25, 3) -> (18.25, 8)
  line L3 (18.25, 8) -> (18.5, 8)
  line L4 (18.5, 8) -> (18.5, 3)
  line L5 (17.5, 3) -> (16.5, 3) projected
  line L6 (18.5, 29.81) -> (18.25, 29.81)
  line L7 (18.25, 29.81) -> (18.25, 34.81)
  line L8 (18.25, 34.81) -> (18.5, 34.81)
  line L9 (18.5, 34.81) -> (18.5, 29.81)
  line L10 (17.5, 29.81) -> (16.5, 29.81) projected
  point P0 (-3, 15.5541)
  point P1 (18.5, 8)
  dimension "d97" = 0.25
  dimension "d98" = 5
  dimension "d99" = 0
  dimension "d100" = 0.25
  dimension "d101" = 5
  dimension "d102" = 0
  constraints: 16 end point, 4 parallel, 2 horizontal, 2 perpendicular, 2 point on line
  measures "d97" distance of L2.end L3.end
  measures "d98" distance of L1.end L2.end
  measures "d99" distance between parallel lines of L5 L1
  measures "d100" distance of L7.end L8.end
  measures "d101" distance of L6.end L7.end
  measures "d102" distance between parallel lines of L10 L6
extrude "Oeffnungskerben1" cut sketch "Sketch23" against normal through all
sketch "Sketch24" plane through (3, 9.0441, -27.7559) normal (0, -1, 0) x (1, 0, 0)
  line L0 (18.5, 22.51) -> (18.5, 0) projected
  line L1 (18.5, 8.5) -> (18.25, 8.5)
  line L2 (18.25, 8.5) -> (18.25, 13.5)
  line L3 (18.25, 13.5) -> (18.5, 13.5)
  line L4 (18.5, 13.5) -> (18.5, 8.5)
  line L5 (17.5, 8.5) -> (16.5, 8.5) projected
  line L6 (18.5, 43.31) -> (18.5, 31.91) projected
  line L7 (18.5, 35.31) -> (18.25, 35.31)
  line L8 (18.25, 35.31) -> (18.25, 40.31)
  line L9 (18.25, 40.31) -> (18.5, 40.31)
  line L10 (18.5, 40.31) -> (18.5, 35.31)
  line L11 (17.5, 35.31) -> (16.5, 35.31) projected
  point P0 (-3, 27.7559)
  dimension "d105" = 0.25
  dimension "d106" = 5
  dimension "d107" = 0
  dimension "d108" = 0.25
  dimension "d109" = 5
  dimension "d110" = 0
  constraints: 16 end point, 4 parallel, 2 horizontal, 2 perpendicular, 2 point on line
  measures "d105" distance of L2.end L3.end
  measures "d106" distance of L1.end L2.end
  measures "d107" distance between parallel lines of L5 L1
  measures "d108" distance of L8.end L9.end
  measures "d109" distance of L7.end L8.end
  measures "d110" distance between parallel lines of L11 L7
extrude "Oeffnugskerben2" cut sketch "Sketch24" against normal through all
equation "\"MinimumRemnant\" = 2 * Thickness"
equation "\"BendRadius\" = Thickness"
equation "\"BendReliefWidth\" = Thickness"
equation "\"BendReliefDepth\" = 0.5 * Thickness"
equation "\"CornerReliefSize\" = 4 * Thickness"
equation "\"TransitionRadius\" = BendRadius"
equation "\"JacobiRadiusSize\" = BendRadius"
equation "\"GapSize\" = Thickness"
equation "\"Thickness\" = 0.5"
body "Solid1"
